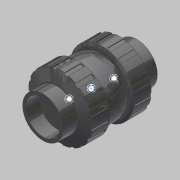
# Autodesk Inventor part: CHECK VALVE TRUE UNION GLUED DN50
Saved by Autodesk Inventor 2017 (Build 210142000, 142)
## iProperties
Created: 2016-04-26
Part Number: CHECK VALVE TRUE UNION GLUED DN50
Description: SXEIV VINK
Document SubType Name: Modeling
Manufacturer: SEKISUI
Mass: 197.859 g
Surface Area: 285.44 cm^2
Volume: 153.379 cm^3
Density: 1.29 g/cm^3
Material: U-PVC
Appearance: Smooth - Medium Gray
Catalog Web Link: http://www.pocketbrewery.com
Title: BALL VALVE PVC-U TRD DN15
Autodesk Inventor part; units mm, degrees
ref_plane "YZ Plane" through (0, 0, 0) normal (1, 0, 0) x (0, 1, 0)
ref_plane "XZ Plane" through (0, 0, 0) normal (0, 1, 0) x (-1, 0, 0)
ref_plane "XY Plane" through (0, 0, 0) normal (0, 0, 1) x (1, 0, 0)
sketch "Sketch_1" plane through (0, 0, 0) normal (0, 0, 1) x (1, 0, 0)
  line L0 (61.5, 0) -> (61.5, -39.3333)
  line L1 (61.5, -39.3333) -> (54.3419, -59)
  line L2 (54.3419, -59) -> (22.3917, -59)
  line L3 (22.3917, -59) -> (20.5, -53.8027)
  line L4 (20.5, -53.8027) -> (20.5, -48.2718)
  arc A0 (-20.5, -48.2718) -> (20.5, -48.2718) centre (0, 0) ccw
  line L5 (-20.5, -48.2718) -> (-20.5, -53.8027)
  line L6 (-20.5, -53.8027) -> (-22.3917, -59)
  line L7 (-22.3917, -59) -> (-54.3419, -59)
  line L8 (-54.3419, -59) -> (-61.5, -39.3333)
  line L9 (-61.5, -39.3333) -> (-61.5, 0)
  line L10 (-61.5, 0) -> (61.5, 0)
  line L11 (-22.3917, -59) -> (0, -59) construction
  line L12 (0, -59) -> (0, -52.4444) construction
  line L13 (-55.0699, -59) -> (-24.3917, -59)
  line L14 (-24.3917, -59) -> (-24.3917, -57)
  line L15 (-24.3917, -57) -> (-55.0699, -57)
  line L16 (-55.0699, -57) -> (-55.0699, -59)
  line L17 (24.3917, -59) -> (55.0699, -59)
  line L18 (55.0699, -59) -> (55.0699, -57)
  line L19 (55.0699, -57) -> (24.3917, -57)
  line L20 (24.3917, -57) -> (24.3917, -59)
  point P0 (-38.3668, -59)
  dimension "dimZ" = 123
  dimension "dimE" = 118
  dimension "d22" = 59
  dimension "d23" = 19.6667
  dimension "d24" = 20
  dimension "d27" = 41
  dimension "d28" = 41
  dimension "d40" = 6.5556
  dimension "d52" = 20
  dimension "d53" = 2
  dimension "d54" = 2
  dimension "d55" = 2
  constraints: 42 end point, 6 parallel, 5 equal length, 5 perpendicular, 4 horizontal, 3 collinear, 3 point on circle, 3 point on line, 2 coincident, 2 midpoint, 1 centre point
  measures "dimZ" distance of L9.end L0.start
  measures "dimE" diameter of L2 L10
  measures "d22" distance from line of L0.start L2
  measures "d23" vertical distance of L0.end L1.end
  measures "d24" angle of L0 L1
  measures "d27" distance between parallel lines of L9 L5
  measures "d28" distance between parallel lines of L0 L4
  measures "d40" distance of L11.end L12.end
  measures "d52" angle of L5 L6
  measures "d53" distance of L15.end L13.start
  measures "d54" distance from line of L6.end L14
  measures "d55" distance from line of L2.end L20
revolve "Revolution1" add sketch "Sketch_1" angle 360 about axis through (-61.5, 0, 0) along (1, 0, 0) contours L0 L1 L19 L20 L2 L3 L4 A0 L5 L6 L7 L14 L15 L8 L9 L10 | L1 L2 L20 L19 | L15 L14 L7 L8
sketch "Sketch_7" plane through (0, 0, 0) normal (0, 0, 1) x (1, 0, 0)
  line L0 (-87, 37.5) -> (87, 37.5)
  line L1 (48.5126, 0) -> (-48.5126, 0)
  line L2 (-87, 37.5) -> (-87, 31.5)
  line L3 (-87, 31.5) -> (87, 31.5)
  line L4 (87, 31.5) -> (87, 37.5)
  line L5 (0, -5) -> (0, 30) projected
  point P0 (0, 0)
  point P1 (0, 0)
  point P2 (0, 31.5)
  dimension "dimH" = 174
  dimension "dimD" = 63
  dimension "dimD2" = 75
  constraints: 10 end point, 2 midpoint, 2 perpendicular, 1 coincident, 1 horizontal, 1 parallel, 1 point on line, 1 vertical
  measures "dimH" distance of L2.end L3.end
  measures "dimD" diameter of L3 L1
  measures "dimD2" diameter of L0 L1
revolve "Revolution3" add sketch "Sketch_7" angle 360 about axis through (48.5126, 0, 0) along (-1, 0, 0)
extrude "Extrusion8" cut sketch "Sketch_1" along normal mid plane 7.8667 contours L18 L17 L1 | L1 L2 L20 L19 | L15 L14 L7 L8 | L8 L13 L16
pattern_circular "Circular Pattern1" count 17 over 360 about axis through (43.5, 0, 0) along (-1, 0, 0) of "Extrusion8"
equation "\"d23\" = 0.333333 * d22"
equation "\"d27\" = 0.333333 * dimZ"
equation "\"d28\" = d27"
equation "\"d40\" = 0.333333 * d23"
equation "\"d47\" = 0.0666667 * dimE"
equation "\"oMe\" = dimE"
body "Solid1"
